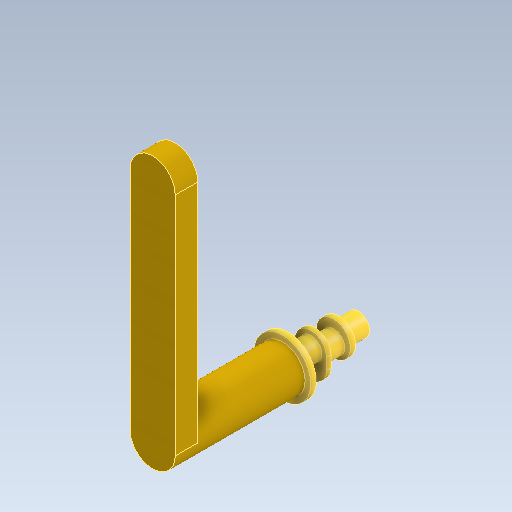
# Autodesk Inventor part: Input Shaft
Saved by Autodesk Inventor 2026.2 (Build 302298010, 298A)
## iProperties
Created: 2026-07-15
Part Number: Input Shaft
Material: Generic
Document SubType Name: Modeling
Designer: maxim
Density: 1 g/cm^3
Appearance: Glossy - Gold
Mass: 41.9651 g
Surface Area: 142.905 cm^2
Volume: 41.9651 cm^3
Author: maxim
Autodesk Inventor part; units mm, degrees
sketch "Sketch1" plane through (0, 0, 0) normal (0, 0, 1) x (1, 0, 0)
  circle A0 centre (0, 0) radius 10
  dimension "d0" = 20
  constraints: 1 centre point, 1 coincident
  measures "d0" diameter of A0
extrude "Extrusion1" add sketch "Sketch1" against normal blind 50
sketch "Sketch2" plane through (0, 0, -50) normal (0, 0, -1) x (-1, 0, 0)
  circle A0 centre (0, 1.25) radius 4.95
  circle A1 centre (0, 1.25) radius 7
  point P0 (0, 0)
  dimension "d3" = 9.9
  dimension "d4" = 1.25
  dimension "d70" = 14
  constraints: 2 centre point, 1 vertical alignment
  measures "d3" diameter of A0
  measures "d4" distance of A0.centre point (0, 0)
  measures "d70" diameter of A1
extrude "Extrusion2" add sketch "Sketch2" along normal blind 10 contours A0
sketch "Sketch4" plane through (0, 1.25, -60) normal (0, 0, -1) x (-1, 0, 0)
  line L0 (0, 0) -> (0, -5) construction
  line L1 (-6.95, 0) -> (-6.95, -5)
  line L2 (6.95, -5) -> (6.95, 0)
  arc A0 (6.95, 0) -> (-6.95, 0) centre (0, 0) ccw
  arc A1 (-6.95, -5) -> (6.95, -5) centre (0, -5) ccw
  circle A2 centre (0, 0) radius 4.95 projected
  circle A3 centre (0, 0) radius 6.95
  point P0 (0, -1.25)
  point P1 (0, -2.5)
  point P2 (-6.95, 0)
  dimension "d12" = 1.25
  dimension "d23" = 2
  dimension "d39" = 2
  dimension "d73" = 1.25
  constraints: 8 end point, 4 point on circle, 4 tangent, 3 centre point, 1 midpoint, 1 parallel, 1 vertical, 1 vertical alignment
  measures "d12" distance of L0.start point (0, -1.25)
  measures "d23" radial gap between concentric circles of A0 A2
  measures "d39" radial gap between concentric circles of A2 A3
  measures "d73" distance of point (0, -2.5) point (0, -1.25)
extrude "Extrusion4" add sketch "Sketch4" along normal blind 2 contours A3 L2 A1 L1 | A0 A3 | A2
sketch "Sketch5" plane through (0, 1.25, -62) normal (0, 0, -1) x (-1, 0, 0)
  circle A0 centre (0, -2.5) radius 4.95
  circle A1 centre (0, -1.25) radius 10 projected
  circle A2 centre (0, -2.5) radius 7
  dimension "d16" = 9.9
  dimension "d17" = 1.25
  dimension "d71" = 14
  constraints: 2 centre point, 1 vertical alignment
  measures "d16" diameter of A0
  measures "d17" distance of A1.centre A0.centre
  measures "d71" diameter of A2
extrude "Extrusion5" add sketch "Sketch5" along normal blind 8.05 contours A0
sketch "Sketch6" plane through (0, 0, 0) normal (0, 0, 1) x (1, 0, 0)
  line L0 (0, 0) -> (0, 100) construction
  line L1 (-10, 0) -> (-10, 100)
  line L2 (10, 100) -> (10, 0)
  arc A0 (-10, 0) -> (10, 0) centre (0, 0) ccw
  arc A1 (10, 100) -> (-10, 100) centre (0, 100) ccw
  point P0 (0, 50)
  dimension "d22" = 10
  dimension "d72" = 100
  constraints: 8 end point, 4 point on circle, 4 tangent, 2 centre point, 1 midpoint, 1 parallel, 1 vertical
  measures "d22" radius of A0
  measures "d72" distance of L0.start L0.end
extrude "Extrusion6" add sketch "Sketch6" along normal blind 10
sketch "Sketch7" plane through (0, 0, -50) normal (0, 0, -1) x (-1, 0, 0)
  circle A0 centre (0, 0) radius 12.5
  dimension "d25" = 25
  constraints: 1 centre point, 1 coincident
  measures "d25" diameter of A0
extrude "Extrusion7" add sketch "Sketch7" against normal blind 2.5
extrude "Extrusion14" add sketch "Sketch2" along normal blind 1.95
ref_plane "Work Plane1" through (0, 1.25, -66.025) normal (0, 0, -1) x (-1, 0, 0)
ref_plane "Work Plane2" through (0, 1.25, -55.975) normal (0, 0, -1) x (-1, 0, 0)
sketch "Sketch10" plane through (0, -1.25, -70.05) normal (0, 0, -1) x (-1, 0, 0)
  circle A0 centre (0, 1.25) radius 7.5
  circle A1 centre (0, 1.25) radius 4.95
  dimension "d49" = 15
  dimension "d52" = 9.9
  constraints: 2 centre point, 2 coincident
  measures "d49" diameter of A0
  measures "d52" diameter of A1
extrude "Extrusion15" add sketch "Sketch10" along normal blind 2.25 contours A0 | A1
extrude "Extrusion16" add sketch "Sketch10" along normal blind 11 contours A1
ref_plane "Work Plane4" through (0, 0, -47.5) normal (0, 0, 1) x (1, 0, 0)
ref_plane "Work Plane5" through (0, 1.25, -60) normal (0, 0, 1) x (1, 0, 0)
ref_plane "Work Plane6" through (0, 0, -70.05) normal (0, 0, 1) x (1, 0, 0)
split body "Split2" result two bodies by plane through (0, 0, -47.5) normal (0, 0, 1) first body at (9.377, -1.5239, -12.5)
split body "Split3" result two bodies by plane through (0, 1.25, -60) normal (0, 0, 1) bodies 3 first body at (-0.2813, -10.1722, -49.5)
split body "Split4" result two bodies by plane through (0, 0, -70.05) normal (0, 0, 1) bodies 5 first body at (-4.4356, -1.6081, -67.3667)
sketch "Sketch11" plane through (0, 0, -47.5) normal (0, 0, -1) x (-1, 0, 0)
  circle A0 centre (0, 0) radius 2.85
  line L0 (-1.2759, -2.5484) -> (-1.2759, 2.5484)
  point P0 (-2.85, 0)
  point P1 (0, 2.85)
  dimension "d62" = 5.7
  constraints: 2 end point, 2 point on circle, 1 centre point, 1 coincident, 1 horizontal alignment, 1 vertical, 1 vertical alignment
  measures "d62" diameter of A0
extrude "Extrusion18" add sketch "Sketch11" along normal blind 34 contours A0 L0 picked at (0.0994, 0) bodies 2
combine bodies "Combine2" operation type subtract main body 4 bodies to subtract 2 keep tools yes
combine bodies "Combine3" operation type subtract main body 6 bodies to subtract 2 keep tools yes
combine bodies "Combine4" operation type subtract main body 7 bodies to subtract 2 keep tools yes
sketch "Sketch12" plane through (0, 0, -81.5) normal (0, 0, -1) x (-1, 0, 0)
  arc A0 (-1.2759, -2.5484) -> (-1.2759, 2.5484) centre (0, 0) ccw projected
  line L0 (-1.2759, 2.5484) -> (-1.2759, -2.5484) projected
  arc A1 (-1.3259, -2.5791) -> (-1.3259, 2.5791) centre (0, 0) ccw
  line L1 (-1.3259, -2.5791) -> (-1.3259, 2.5791)
  dimension "d65" = 0.05
  constraints: 2 end point, 2 point on circle, 1 centre point, 1 other
  measures "d65" distance between parallel lines of L0 L1
extrude "Extrusion20" cut sketch "Sketch12" against normal up to surface (34 mm away) bodies 2 7 6 4
body "Solid4"
body "Solid6"
body "Solid8"
body "Solid9"
